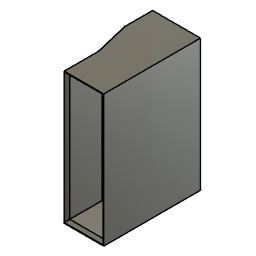
Inverter_fan_cabinet_vertical (Autodesk Fusion 360 design; units mm, degrees)
Autodesk Fusion 360 part; units mm, degrees
sketch "Sketch1" plane through (0, 0, 0) normal (0, 1, 0) x (1, 0, 0)
  line L0 (0, 0) -> (70, 0)
  line L1 (70, 0) -> (70, -40)
  line L2 (0, -40) -> (0, 0)
  line L3 (70, -40) -> (12, -40)
  line L4 (70, -90) -> (70, -40)
  line L5 (0, -40) -> (12, -90)
  line L6 (12, -90) -> (12, -140)
  line L7 (12, -140) -> (70, -140)
  line L8 (70, -140) -> (70, -90)
  dimension "d1" = 70
  dimension "d2" = 40
  dimension "d3" = 58
  dimension "d4" = 50
  dimension "d5" = 58
  dimension "d6" = 50
  constraint horizontal L0
  constraint vertical L1
  constraint vertical L2
  constraint coincident L0.start L2.end
  constraint horizontal L3
  constraint vertical L4
  constraint vertical L6
  constraint horizontal L7
  constraint vertical L8
  measures "d1" distance of L0.start L0.end
  measures "d2" distance of L0.start L2.start
  measures "d3" distance of L1.end L3.end
  measures "d4" distance of L1.end L4.start
  measures "d5" distance of L4.start L5.end
  measures "d6" distance of L4.start L7.end
extrude "Extrude1" add sketch "Sketch1" along normal blind 190
sketch "Sketch2" plane through (0, 0, 0) normal (0, 0, -1) x (-1, 0, 0)
  line L0 (-70, 0) -> (0, 0)
  line L1 (0, 0) -> (0, 190)
  line L2 (0, 190) -> (-70, 190)
  line L3 (-70, 190) -> (-70, 0)
sketch "Sketch4" plane through (0, 0, 0) normal (0, 0, -1) x (-1, 0, 0)
  circle A0 centre (-35, 155) radius 25
  line L0 (0, 190) -> (-70, 190)
  line L1 (0, 0) -> (0, 190)
  circle A1 centre (-35, 95) radius 25
  circle A2 centre (-35, 35) radius 25
  dimension "d21" = 50
  dimension "d22" = 35
  dimension "d23" = 35
  dimension "d24" = 50
  dimension "d25" = 35
  dimension "d26" = 60
  dimension "d27" = 50
  dimension "d28" = 35
  dimension "d29" = 60
  measures "d21" diameter of A0
  measures "d22" distance of A0.centre L0
  measures "d23" distance of A0.centre L1
  measures "d24" diameter of A1
  measures "d25" distance of L1 A1.centre
  measures "d26" distance of A0.centre A1.centre
  measures "d27" diameter of A2
  measures "d28" distance of L1 A2.centre
  measures "d29" distance of A1.centre A2.centre
shell "Shell1" thickness 5 removed faces 1 at (31.3333, 63.3333, 140)
extrude "Extrude2" cut sketch "Sketch4" against normal blind 25
fillet "Fillet1" radius 1 7 edges at (12, 190, 115) (6, 190, 65) (0, 190, 20) (12, 95, 140) (12, 0, 115) (6, 0, 65) (0, 0, 20)
fillet "Fillet2" radius 1 3 edges at (0.2929, 0.2929, 39.9653) (0, 95, 40) (0.2929, 189.7071, 39.9653)
chamfer "Chamfer1" distance 4 angle 45 4 edges at (65, 95, 140) (41, 185, 140) (17, 95, 140) (41, 5, 140)
fillet "Fillet3" radius 0.5 6 edges at (70, 95, 0) (35.5, 190, 0) (0.2929, 189.7071, 0) (0, 95, 0) (0.2929, 0.2929, 0) (35.5, 0, 0)
